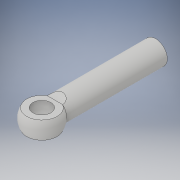
# Autodesk Inventor part: Ball Joint Female
Saved by Autodesk Inventor 2018.2 (Build 222227000, 227)
## iProperties
Created: 2018-02-18
Part Number: Ball Joint Female
Material: Generisch
Document SubType Name: Modeling
Designer: JochenAlt
Density: 1 g/cm^3
Appearance: Vorgabe
Author: JochenAlt
Autodesk Inventor part; units mm, degrees
ref_plane "YZ Plane" through (0, 0, 0) normal (1, 0, 0) x (0, 1, 0)
ref_plane "XZ Plane" through (0, 0, 0) normal (0, 1, 0) x (-1, 0, 0)
ref_plane "XY Plane" through (0, 0, 0) normal (0, 0, 1) x (1, 0, 0)
sketch "Skizze1" plane through (0, 0, 0) normal (0, 0, 1) x (1, 0, 0)
  line L0 (-14, 0) -> (14, 0) construction
  line L1 (0, 36.2472) -> (0, -10.9833) construction
  arc A0 (0, -2.15) -> (0, 2.15) centre (0, 0) ccw
  arc A1 (0, -3) -> (2, 2.2361) centre (0, 0) ccw
  line L2 (2, 2.2361) -> (2, 19.5)
  line L3 (2, 19.5) -> (1.2, 19.5)
  line L4 (0, 3.15) -> (0, 2.15)
  line L5 (0, -2.15) -> (0, -3)
  line L6 (-10, -4.2361) -> (10, -4.2361)
  line L7 (10, -4.2361) -> (10, 4.2361)
  line L8 (10, 4.2361) -> (-10, 4.2361)
  line L9 (-10, 4.2361) -> (-10, -4.2361)
  line L10 (-10, -4.2361) -> (10, 4.2361) construction
  line L11 (10, -4.2361) -> (-10, 4.2361) construction
  line L12 (0, 3.15) -> (1.2, 3.15)
  line L13 (1.2, 19.5) -> (1.2, 3.15)
  line L14 (-10, 4.2361) -> (-10, 29.5)
  line L15 (-10, 29.5) -> (10, 29.5)
  line L16 (10, 29.5) -> (10, 4.2361)
  point P0 (0, 15)
  dimension "d1" = 4.3
  dimension "d2" = 6
  dimension "d6" = 19.5
  dimension "d7" = 10
  dimension "d11" = 1
  dimension "d12" = 1.2
  dimension "d13" = 0.8
  dimension "d19" = 2
  dimension "d22" = 10
  constraints: 30 end point, 5 perpendicular, 5 point on line, 4 point on circle, 3 midpoint, 3 vertical, 2 centre point, 2 parallel, 1 coincident, 1 horizontal
  measures "d1" diameter of A0
  measures "d2" diameter of A1
  measures "d6" distance between parallel lines of L3 L0
  measures "d7" distance between parallel lines of L7 L1
  measures "d11" distance of L4.end L4.start
  measures "d12" distance between parallel lines of L13 L1
  measures "d13" distance between parallel lines of L2 L13
  measures "d19" distance from line of L8 L2.start
  measures "d22" distance between parallel lines of L15 L3
revolve "Umdrehung1" add sketch "Skizze1" angle 360 about axis through (0, 0, 0) along (0, -1, 0) contours A0 L4 L12 L13 L8 L2 A1 L5 | L8 L13 L3 L2
extrude "Extrusion1" add sketch "Skizze1" along normal mid plane 3 separate body contours L5 A1 L2 L8 L7 L6 L9 L13 L12 L4 A0 | A0 L4 L12 L13 L8 L2 A1 L5
extrude "Extrusion2" add sketch "Skizze1" along normal mid plane 20 contours L8 L13 L3 L2 | L2 L3 L13 L8 L14 L15 L16 bodies 2
fillet "Rundung1" radius 2 2 edges at (0, 4.2361, -1.5) (0, 4.2361, 1.5)
combine bodies "Kombinieren1" operation type common bodies to combine 1 2
thread "Gewinde2" size "M2.5x0.45" class "6H" standard "ANSI Metric M Profile" full length
